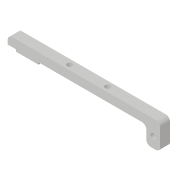
# Autodesk Inventor part: PhoneMountRightRib
Saved by Autodesk Inventor 2018 (Build 220112000, 112)
## iProperties
Created: 2019-02-13
Part Number: PhoneMountRightRib
Material: Generic
Document SubType Name: Modeling
Designer: ball
Density: 1 g/cm^3
Appearance: Default
Author: ball
Autodesk Inventor part; units mm, degrees
ref_plane "YZ Plane" through (0, 0, 0) normal (1, 0, 0) x (0, 1, 0)
ref_plane "XZ Plane" through (0, 0, 0) normal (0, 1, 0) x (-1, 0, 0)
ref_plane "XY Plane" through (0, 0, 0) normal (0, 0, 1) x (1, 0, 0)
ref_plane "Work Plane1" through (65.1649, 36.0099, -59.025) normal (0, 0, -1) x (0, -1, 0)
ref_plane "Work Plane2" through (0, 0, 0) normal (0, 0, 1) x (1, 0, 0)
sketch "Sketch1" plane through (0, 0, 0) normal (0, 0, 1) x (1, 0, 0)
  line L0 (27.0649, 36.0099) -> (65.1649, 36.0099) construction
  line L1 (-10, 0) -> (-10, 27.6599) construction
  line L2 (102.2297, 27.6599) -> (102.2297, 0) construction
  line L3 (89.2297, 29.6599) -> (100.2297, 29.6599) construction
  line L4 (-10, 36.0099) -> (102.2297, 36.0099)
  line L5 (102.2297, 36.0099) -> (102.2297, 29.6599)
  line L6 (92.075, 29.6599) -> (-10, 29.6599)
  line L7 (-10, 29.6599) -> (-10, 36.0099)
  line L8 (92.075, 29.6599) -> (92.075, 16.9599)
  line L9 (92.075, 16.9599) -> (102.2297, 16.9599)
  line L10 (102.2297, 16.9599) -> (102.2297, 29.6599)
  circle A0 centre (97.2297, 24.6599) radius 1.965 projected
  circle A1 centre (97.2297, 24.6599) radius 1.965 construction
  point P0 (0, 0)
  constraints: 14 end point, 3 parallel, 1 horizontal, 1 perpendicular, 1 point on line
extrude "Extrusion1" add sketch "Sketch1" along normal blind 7.366
fillet "Fillet1" radius 3.175 4 edges at (92.075, 29.6599, 3.683) (102.2297, 36.0099, 3.683) (92.075, 16.9599, 3.683) (102.2297, 16.9599, 3.683)
sketch "Sketch2" plane through (0, 0, 0) normal (0, 0, -1) x (-1, 0, 0)
  line L0 (10, 0) -> (10, 27.6599) construction
  line L1 (-88.9, 29.6599) -> (10, 29.6599) projected
  line L2 (10, 29.6599) -> (-6.51, 29.6599)
  line L3 (-6.51, 29.6599) -> (-6.51, 22.0399)
  line L4 (-6.51, 22.0399) -> (10, 22.0399)
  line L5 (10, 22.0399) -> (10, 29.6599)
  point P0 (0, 0)
  dimension "d4" = 16.51
  dimension "d5" = 7.62
  constraints: 10 end point, 2 parallel, 1 horizontal, 1 perpendicular, 1 vertical, 2 other
  measures "d4" distance of L4.end L3.end
  measures "d5" distance of L3.end L2.end
extrude "Extrusion2" add sketch "Sketch2" against normal blind 1.27
fillet "Fillet2" radius 1.524 1 edges at (-1.745, 29.6599, 1.27)
sketch "Sketch3" plane through (0, 0, 0) normal (0, 0, -1) x (-1, 0, 0)
  circle A0 centre (5, 24.6599) radius 1.965 construction
  arc A1 (6.5875, 24.6599) -> (3.4125, 24.6599) centre (5, 24.6599) ccw
  line L0 (3.4125, 24.6599) -> (6.5875, 24.6599)
  point P0 (0, 0)
  dimension "d9" = 3.175
  constraints: 2 centre point, 2 end point, 2 point on circle, 1 coincident, 2 other
  measures "d9" diameter of A1
revolve "Revolution1" add sketch "Sketch3" angle 180 about axis through (-3.4125, 24.6599, 0) along (-1, 0, 0)
sketch "Sketch4" plane through (-10, 29.6599, 7.366) normal (0, -1, 0) x (1, 0, 0)
  line L0 (37.0649, -133.32) -> (37.0649, 0.03) construction
  line L1 (75.1649, 0.03) -> (75.1649, -133.32) construction
  line L2 (0, 0) -> (98.9, 0) construction
  line L3 (109.0547, 0) -> (0, 0) construction
  line L4 (37.0649, 0) -> (37.0649, -7.366) construction
  line L5 (0, -7.366) -> (109.0547, -7.366) construction
  line L6 (75.1649, 0) -> (75.1649, -7.366) construction
  line L7 (37.0649, -3.683) -> (75.1649, -3.683) construction
  point P0 (10, -7.366)
  point P1 (42.1449, -3.683)
  point P2 (70.0849, -3.683)
  dimension "d11" = 5.08
  dimension "d12" = 5.08
  constraints: 10 end point, 10 point on line, 2 midpoint, 2 vertical, 4 other
  measures "d11" distance from line of point (42.145, -3.683) L0
  measures "d12" distance from line of point (70.085, -3.683) L1
hole "Hole1" at (32.1449, 29.6599, 3.683) at (60.0849, 29.6599, 3.683) direction (0, 1, 0) diameter 3.937 end through all
fillet "Fillet3" radius 3.175 1 edges at (-10, 36.0099, 3.683)
fillet "Fillet4" radius 1.524 1 edges at (6.51, 29.6599, 1.397)
body "Solid1"
